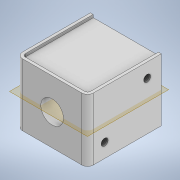
# Autodesk Inventor part: main_block
Saved by Autodesk Inventor 2021 (Build 250183000, 183)
## iProperties
Created: 2020-06-26
Part Number: main_block
Material: Generic
Document SubType Name: Modeling
Designer: Yatekii
Density: 1 g/cm^3
Appearance: Default
Author: Yatekii
Autodesk Inventor part; units mm, degrees
ref_plane "YZ Plane" through (0, 0, 0) normal (1, 0, 0) x (0, 1, 0)
ref_plane "XY Plane" through (0, 0, 0) normal (0, 0, 1) x (1, 0, 0)
sketch "Sketch2" plane through (0, 0, 0) normal (0, 1, 0) x (-1, 0, 0)
  line L0 (-12.5, -13) -> (12.5, -13)
  line L1 (12.5, -13) -> (12.5, 13)
  line L2 (12.5, 13) -> (-12.5, 13)
  line L3 (-12.5, 13) -> (-12.5, -13)
  line L4 (-12.5, -13) -> (12.5, 13) construction
  line L5 (12.5, -13) -> (-12.5, 13) construction
  point P0 (0, 0)
  dimension "d0" = 25
  dimension "d1" = 26
  constraints: 12 end point, 2 midpoint, 2 parallel, 1 horizontal, 1 perpendicular
  measures "d0" distance of L2.end L1.end
  measures "d1" distance of L1.end L0.end
extrude "Extrusion1" add sketch "Sketch2" along normal blind 22
sketch "Sketch3" plane through (12.5, 0, 13) normal (1, 0, 0) x (0, 0, -1)
  line L0 (0, 0) -> (26, 0) projected
  line L1 (0, 22) -> (26, 22) projected
  line L2 (0, 0) -> (0, 22) projected
  point P0 (13, 0)
  point P1 (6, 5)
  point P2 (21, 17)
  dimension "d4" = 12
  dimension "d5" = 5
  dimension "d6" = 5
  dimension "d7" = 6
  dimension "d8" = 15
  measures "d4" vertical distance of point (21, 17) point (6, 5)
  measures "d5" distance from line of L0 point (6, 5)
  measures "d6" distance from line of L1 point (21, 17)
  measures "d7" distance from line of L2 point (6, 5)
  measures "d8" horizontal distance of point (21, 17) point (6, 5)
hole "Hole1" at (12.5, 5, 7) at (12.5, 17, -8) direction (-1, 0, 0) diameter 2.459 depth 8.8 thread size "M3x0.5" class "6H" standard "ISO Metric profile"
mirror "Mirror1" about plane through (0, 0, 0) normal (1, 0, 0) of "Hole1"
fillet "Fillet1" radius 2 2 edges at (12.5, 11, 13) (-12.5, 11, 13)
sketch "Sketch4" plane through (0, 22, 0) normal (0, 1, 0) x (1, 0, 0)
  arc A0 (-12.5, -11) -> (-10.5, -13) centre (-10.5, -11) ccw construction
  line L0 (-10.5, -13) -> (10.5, -13) construction
  arc A1 (10.5, -13) -> (12.5, -11) centre (10.5, -11) ccw construction
  line L1 (12.5, -11) -> (12.5, 13) construction
  line L2 (12.5, 13) -> (-12.5, 13) construction
  line L3 (-12.5, 13) -> (-12.5, -11) construction
  arc A2 (-11.5, -11) -> (-10.5, -12) centre (-10.5, -11) ccw
  line L4 (-10.5, -12) -> (10.5, -12)
  arc A3 (10.5, -12) -> (11.5, -11) centre (10.5, -11) ccw
  line L5 (11.5, -11) -> (11.5, 12)
  line L6 (11.5, 12) -> (-11.5, 12)
  line L7 (-11.5, 12) -> (-11.5, -11)
  line L8 (12.5, 13) -> (-12.5, 13) projected
  line L9 (-11.5, 12) -> (11.5, 12)
  line L10 (11.5, 12) -> (11.5, 13)
  line L11 (11.5, 13) -> (-11.5, 13)
  line L12 (-11.5, 13) -> (-11.5, 12)
  point P0 (0, 0)
  dimension "d17" = 1
  constraints: 16 end point, 4 point on circle, 2 centre point, 2 parallel, 1 horizontal, 1 perpendicular, 1 point on line, 5 other
  measures "d17" distance between parallel lines of L3 L7
extrude "Extrusion2" cut sketch "Sketch4" against normal blind 1
ref_plane "Work Plane1" through (0, 11, 0) normal (0, 1, 0) x (-1, 0, 0)
mirror "Mirror2" about plane through (0, 11, 0) normal (0, 1, 0) of "Extrusion2"
sketch "Sketch5" plane through (-12.5, 0, -13) normal (0, 0, -1) x (-1, 0, 0)
  line L0 (-25, 0) -> (-25, 22) construction
  line L1 (0, 0) -> (0, 22) construction
  line L2 (-25, 0) -> (0, 22) construction
  line L3 (-25, 22) -> (-24, 22) construction
  line L4 (-25, 22) -> (0, 0) construction
  circle A0 centre (-12.5, 11) radius 8
  point P0 (-12.5, 0)
  dimension "d21" = 16
  constraints: 4 end point, 1 centre point, 1 midpoint
  measures "d21" diameter of A0
extrude "Extrusion3" add sketch "Sketch5" along normal blind 2
sketch "Sketch6" plane through (0, 11, -15) normal (0, 0, -1) x (-1, 0, 0)
  circle A0 centre (0, 0) radius 4
  point P0 (0, -11)
  dimension "d24" = 8
  constraints: 1 centre point
  measures "d24" diameter of A0
extrude "Extrusion4" cut sketch "Sketch6" against normal through all
equation "\"d5\" = d6"
body "Solid1"
